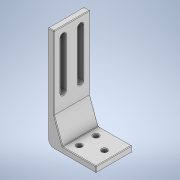
# Autodesk Inventor part: angle
Saved by Autodesk Inventor 2022 (Build 260153000, 153)
## iProperties
Created: 2022-02-23
Part Number: angle
Material: Generic
Document SubType Name: Modeling
Designer: Frey
Density: 1 g/cm^3
Appearance: Default
Author: Frey
Autodesk Inventor part; units mm, degrees
ref_plane "YZ Plane" through (0, 0, 0) normal (1, 0, 0) x (0, 1, 0)
ref_plane "XZ Plane" through (0, 0, 0) normal (0, 1, 0) x (-1, 0, 0)
ref_plane "XY Plane" through (0, 0, 0) normal (0, 0, 1) x (1, 0, 0)
sketch "Sketch1" plane through (0, 0, 0) normal (0, 1, 0) x (-1, 0, 0)
  line L0 (20, 15) -> (-20, 15)
  line L1 (-20, 15) -> (-20, -15)
  line L2 (-20, -15) -> (20, -15)
  line L3 (20, -15) -> (20, 15)
  line L4 (20, 15) -> (-20, -15) construction
  line L5 (-20, 15) -> (20, -15) construction
  point P0 (0, 0)
  point P1 (0, 0)
  point P2 (0, 0)
  dimension "d0" = 30
  dimension "d1" = 40
  constraints: 13 end point, 2 midpoint, 2 parallel, 1 coincident, 1 horizontal, 1 perpendicular
  measures "d0" distance of L0.end L1.end
  measures "d1" distance of L2.end L1.end
extrude "Extrusion1" add sketch "Sketch1" along normal blind 5
sketch "Sketch2" plane through (0, 5, 0) normal (0, 1, 0) x (1, 0, 0)
  line L0 (-20, 15) -> (-20, -15) projected
  line L1 (-20, -15) -> (-15, -15)
  line L2 (-15, -15) -> (-15, 15)
  line L3 (-15, 15) -> (-20, 15)
  line L4 (-20, 15) -> (-20, -15)
  point P0 (0, 0)
  dimension "d4" = 5
  constraints: 8 end point, 2 parallel, 1 horizontal, 1 perpendicular, 1 point on line
  measures "d4" distance between parallel lines of L2 L0
extrude "Extrusion2" add sketch "Sketch2" along normal blind 80
sketch "Sketch3" plane through (-15, 5, 15) normal (1, 0, 0) x (0, 0, -1)
  line L0 (7.75, 72.25) -> (7.75, 32.25) construction
  line L1 (5.5, 72.25) -> (5.5, 32.25)
  line L2 (10, 32.25) -> (10, 72.25)
  arc A0 (10, 72.25) -> (5.5, 72.25) centre (7.75, 72.25) ccw
  arc A1 (5.5, 32.25) -> (10, 32.25) centre (7.75, 32.25) ccw
  line L3 (22.25, 72.25) -> (22.25, 32.25) construction
  line L4 (20, 72.25) -> (20, 32.25)
  line L5 (24.5, 32.25) -> (24.5, 72.25)
  arc A2 (24.5, 72.25) -> (20, 72.25) centre (22.25, 72.25) ccw
  arc A3 (20, 32.25) -> (24.5, 32.25) centre (22.25, 32.25) ccw
  line L6 (0, 0) -> (0, 80) projected
  line L7 (0, 80) -> (30, 80) projected
  point P0 (15, -5)
  point P1 (7.75, 52.25)
  point P2 (22.25, 52.25)
  dimension "d7" = 4.5
  dimension "d8" = 40
  dimension "d9" = 4.5
  dimension "d10" = 40
  dimension "d11" = 14.5
  dimension "d12" = 7.75
  dimension "d13" = 7.75
  constraints: 16 end point, 8 point on circle, 8 tangent, 4 centre point, 2 midpoint, 2 parallel, 2 vertical, 1 horizontal alignment
  measures "d7" distance between parallel lines of L2 L1
  measures "d8" distance of L0.end L0.start
  measures "d9" distance between parallel lines of L5 L4
  measures "d10" distance of L3.end L3.start
  measures "d11" distance of point (22.25, 52.25) point (7.75, 52.25)
  measures "d12" distance from line of L6 point (7.75, 52.25)
  measures "d13" distance from line of L0.start L7
extrude "Extrusion3" cut sketch "Sketch3" against normal up to surface (5 mm away)
sketch "Sketch4" plane through (0, 5, 0) normal (0, 1, 0) x (1, 0, 0)
  circle A0 centre (-2, -7) radius 2
  circle A1 centre (-2, 7) radius 2
  circle A2 centre (12, 0) radius 2
  line L0 (-15, -15) -> (20, -15) projected
  line L1 (20, -15) -> (20, 15) projected
  point P0 (0, 0)
  dimension "d16" = 4
  dimension "d17" = 4
  dimension "d18" = 4
  dimension "d19" = 14
  dimension "d20" = 8
  dimension "d21" = 14
  dimension "d22" = 8
  constraints: 3 centre point, 1 horizontal alignment, 1 vertical alignment
  measures "d16" diameter of A0
  measures "d17" diameter of A1
  measures "d18" diameter of A2
  measures "d19" distance of A1.centre A0.centre
  measures "d20" distance from line of L0 A0.centre
  measures "d21" horizontal distance of A2.centre A1.centre
  measures "d22" distance from line of L1 A2.centre
extrude "Extrusion4" cut sketch "Sketch4" against normal up to surface (5 mm away)
chamfer "Chamfer1" distance 7 angle 70 1 edges at (-15, 5, 0) measured on face at (-11.257, 5, 2.0235)
fillet "Fillet4" radius 0.5 41 edges at (-15, 79.5, -7.25) (-15, 57.25, -9.5) (-15, 35, -7.25) (-15, 57.25, -5) (-15, 79.5, 7.25) (-15, 57.25, 5) (-15, 35, 7.25) (-15, 57.25, 9.5) (-11.5, 14.6162, 15) (6, 5, 15) (-15, 54.6162, 15) (-11.5, 14.6162, -15) (6, 5, -15) (-15, 54.6162, -15) (-20, 42.5, -15) (-20, 42.5, 15) (0, 0, 15) (0, 0, -15) (20, 2.5, -15) (20, 2.5, 15) (20, 5, 0) (20, 0, 0) (-15, 85, 0) (-20, 85, 0) (-20, 79.5, 7.25) (-20, 57.25, 9.5) (-20, 35, 7.25) (-20, 57.25, 5) (-20, 79.5, -7.25) (-20, 57.25, -5) (-20, 35, -7.25) (-20, 57.25, -9.5) (10, 5, 0) (-4, 5, 7) (-4, 5, -7) (-4, 0, -7) (-4, 0, 7) (10, 0, 0) (-17.5, 85, 15) (-17.5, 85, -15) (-8, 5, 0)
fillet "Fillet5" radius 5 3 edges at (-19.8536, 0.1464, 14.8536) (-19.8536, 0.1464, -14.8536) (-20, 0, 0)
body "Solid1"
